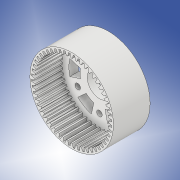
# Autodesk Inventor part: Basespline
Saved by Autodesk Inventor 2017 SP1 (Build 210196100, 196)
## iProperties
Created: 2017-07-11
Part Number: Basespline
Material: ABS Plastic
Document SubType Name: Modeling
Designer: zallen
Density: 1.06 g/cm^3
Appearance: CR White
Author: zallen
Autodesk Inventor part; units mm, degrees
ref_plane "YZ Plane" through (0, 0, 0) normal (1, 0, 0) x (0, 1, 0)
ref_plane "XZ Plane" through (0, 0, 0) normal (0, 1, 0) x (-1, 0, 0)
ref_plane "XY Plane" through (0, 0, 0) normal (0, 0, 1) x (1, 0, 0)
sketch "Sketch1" plane through (0, 0, 0) normal (0, 0, 1) x (1, 0, 0)
  circle A0 centre (0, 0) radius 30 construction
  circle A1 centre (0, 0) radius 33 construction
  circle A2 centre (0, 0) radius 33.1 construction
  circle A3 centre (0, 0) radius 36.1
  line L0 (0, 0) -> (73.8871, 0) construction
  circle A4 centre (0, 0) radius 37.5
  arc A5 (33.0946, -0.6) -> (36.0728, -1.4) centre (38.4543, 13.4097) ccw
  arc A6 (33.0946, 0.6) -> (33.0946, -0.6) centre (53.0856, 0) ccw
  arc A7 (36.0728, 1.4) -> (33.0946, 0.6) centre (38.4543, -13.4097) ccw
  arc A8 (36.0728, -1.4) -> (36.0728, 1.4) centre (0, 0) ccw
  circle A9 centre (0, 0) radius 36.1
  arc A10 (32.9256, 3.3935) -> (35.9786, 2.9583) centre (36.5576, 17.9471) ccw
  arc A11 (35.6411, 5.7379) -> (32.7809, 4.5847) centre (39.7903, -8.6768) ccw
  arc A12 (35.9786, 2.9583) -> (35.6411, 5.7379) centre (0, 0) ccw
  arc A13 (32.7809, 4.5847) -> (32.9256, 3.3935) centre (52.6985, 6.3988) ccw
  circle A14 centre (0, 0) radius 36.1
  arc A15 (32.2765, 7.3375) -> (35.3597, 7.2735) centre (34.1277, 22.2228) ccw
  arc A16 (34.6896, 9.9921) -> (31.9893, 8.5026) centre (40.5461, -3.8174) ccw
  arc A17 (35.3597, 7.2735) -> (34.6896, 9.9921) centre (0, 0) ccw
  arc A18 (31.9893, 8.5026) -> (32.2765, 7.3375) centre (51.543, 12.7042) ccw
  circle A19 centre (0, 0) radius 36.1
  arc A20 (31.1567, 11.1745) -> (34.2251, 11.4826) centre (31.2003, 26.1744) ccw
  arc A21 (33.2322, 14.1006) -> (30.7312, 12.2965) centre (40.7106, 1.0978) ccw
  arc A22 (34.2251, 11.4826) -> (33.2322, 14.1006) centre (0, 0) ccw
  arc A23 (30.7312, 12.2965) -> (31.1567, 11.1745) centre (49.6359, 18.8244) ccw
  circle A24 centre (0, 0) radius 36.1
  arc A25 (29.5826, 14.8485) -> (32.5915, 15.5242) centre (27.8178, 29.7444) ccw
  arc A26 (31.2903, 18.0035) -> (29.0249, 15.9111) centre (40.2814, 5.9969) ccw
  arc A27 (32.5915, 15.5242) -> (31.2903, 18.0035) centre (0, 0) ccw
  arc A28 (29.0249, 15.9111) -> (29.5826, 14.8485) centre (47.0049, 24.6701) ccw
  circle A29 centre (0, 0) radius 36.1
  arc A30 (27.5771, 18.3061) -> (30.4827, 19.3395) centre (24.0297, 32.8805) ccw
  arc A31 (28.8921, 21.6439) -> (26.8955, 19.2936) centre (39.2649, 10.8085) ccw
  arc A32 (30.4827, 19.3395) -> (28.8921, 21.6439) centre (0, 0) ccw
  arc A33 (26.8955, 19.2936) -> (27.5771, 18.3061) centre (43.6886, 30.156) ccw
  circle A34 centre (0, 0) radius 36.1
  arc A35 (25.1695, 21.4966) -> (27.9293, 22.8728) centre (19.8912, 35.5373) ccw
  arc A36 (26.0725, 24.9686) -> (24.3738, 22.3949) centre (37.6758, 15.4626) ccw
  arc A37 (27.9293, 22.8728) -> (26.0725, 24.9686) centre (0, 0) ccw
  arc A38 (24.3738, 22.3949) -> (25.1695, 21.4966) centre (39.7351, 35.2022) ccw
  circle A39 centre (0, 0) radius 36.1
  arc A40 (22.3949, 24.3738) -> (24.9686, 26.0725) centre (15.4626, 37.6758) ccw
  arc A41 (22.8728, 27.9293) -> (21.4966, 25.1695) centre (35.5373, 19.8912) ccw
  arc A42 (24.9686, 26.0725) -> (22.8728, 27.9293) centre (0, 0) ccw
  arc A43 (21.4966, 25.1695) -> (22.3949, 24.3738) centre (35.2022, 39.7351) ccw
  circle A44 centre (0, 0) radius 36.1
  arc A45 (19.2936, 26.8955) -> (21.6439, 28.8921) centre (10.8085, 39.2649) ccw
  arc A46 (19.3395, 30.4827) -> (18.3061, 27.5771) centre (32.8805, 24.0297) ccw
  arc A47 (21.6439, 28.8921) -> (19.3395, 30.4827) centre (0, 0) ccw
  arc A48 (18.3061, 27.5771) -> (19.2936, 26.8955) centre (30.156, 43.6886) ccw
  circle A49 centre (0, 0) radius 36.1
  arc A50 (15.9111, 29.0249) -> (18.0035, 31.2903) centre (5.9969, 40.2814) ccw
  arc A51 (15.5242, 32.5915) -> (14.8485, 29.5826) centre (29.7444, 27.8178) ccw
  arc A52 (18.0035, 31.2903) -> (15.5242, 32.5915) centre (0, 0) ccw
  arc A53 (14.8485, 29.5826) -> (15.9111, 29.0249) centre (24.6701, 47.0049) ccw
  circle A54 centre (0, 0) radius 36.1
  arc A55 (12.2965, 30.7312) -> (14.1006, 33.2322) centre (1.0978, 40.7106) ccw
  arc A56 (11.4826, 34.2251) -> (11.1745, 31.1567) centre (26.1744, 31.2003) ccw
  arc A57 (14.1006, 33.2322) -> (11.4826, 34.2251) centre (0, 0) ccw
  arc A58 (11.1745, 31.1567) -> (12.2965, 30.7312) centre (18.8244, 49.6359) ccw
  circle A59 centre (0, 0) radius 36.1
  arc A60 (8.5026, 31.9893) -> (9.9921, 34.6896) centre (-3.8174, 40.5461) ccw
  arc A61 (7.2735, 35.3597) -> (7.3375, 32.2765) centre (22.2228, 34.1277) ccw
  arc A62 (9.9921, 34.6896) -> (7.2735, 35.3597) centre (0, 0) ccw
  arc A63 (7.3375, 32.2765) -> (8.5026, 31.9893) centre (12.7042, 51.543) ccw
  circle A64 centre (0, 0) radius 36.1
  arc A65 (4.5847, 32.7809) -> (5.7379, 35.6411) centre (-8.6768, 39.7903) ccw
  arc A66 (2.9583, 35.9786) -> (3.3935, 32.9256) centre (17.9471, 36.5576) ccw
  arc A67 (5.7379, 35.6411) -> (2.9583, 35.9786) centre (0, 0) ccw
  arc A68 (3.3935, 32.9256) -> (4.5847, 32.7809) centre (6.3988, 52.6985) ccw
  circle A69 centre (0, 0) radius 36.1
  arc A70 (0.6, 33.0946) -> (1.4, 36.0728) centre (-13.4097, 38.4543) ccw
  arc A71 (-1.4, 36.0728) -> (-0.6, 33.0946) centre (13.4097, 38.4543) ccw
  arc A72 (1.4, 36.0728) -> (-1.4, 36.0728) centre (0, 0) ccw
  arc A73 (-0.6, 33.0946) -> (0.6, 33.0946) centre (0, 53.0856) ccw
  circle A74 centre (0, 0) radius 36.1
  arc A75 (-3.3935, 32.9256) -> (-2.9583, 35.9786) centre (-17.9471, 36.5576) ccw
  arc A76 (-5.7379, 35.6411) -> (-4.5847, 32.7809) centre (8.6768, 39.7903) ccw
  arc A77 (-2.9583, 35.9786) -> (-5.7379, 35.6411) centre (0, 0) ccw
  arc A78 (-4.5847, 32.7809) -> (-3.3935, 32.9256) centre (-6.3988, 52.6985) ccw
  circle A79 centre (0, 0) radius 36.1
  arc A80 (-7.3375, 32.2765) -> (-7.2735, 35.3597) centre (-22.2228, 34.1277) ccw
  arc A81 (-9.9921, 34.6896) -> (-8.5026, 31.9893) centre (3.8174, 40.5461) ccw
  arc A82 (-7.2735, 35.3597) -> (-9.9921, 34.6896) centre (0, 0) ccw
  arc A83 (-8.5026, 31.9893) -> (-7.3375, 32.2765) centre (-12.7042, 51.543) ccw
  circle A84 centre (0, 0) radius 36.1
  arc A85 (-11.1745, 31.1567) -> (-11.4826, 34.2251) centre (-26.1744, 31.2003) ccw
  arc A86 (-14.1006, 33.2322) -> (-12.2965, 30.7312) centre (-1.0978, 40.7106) ccw
  arc A87 (-11.4826, 34.2251) -> (-14.1006, 33.2322) centre (0, 0) ccw
  arc A88 (-12.2965, 30.7312) -> (-11.1745, 31.1567) centre (-18.8244, 49.6359) ccw
  circle A89 centre (0, 0) radius 36.1
  arc A90 (-14.8485, 29.5826) -> (-15.5242, 32.5915) centre (-29.7444, 27.8178) ccw
  arc A91 (-18.0035, 31.2903) -> (-15.9111, 29.0249) centre (-5.9969, 40.2814) ccw
  arc A92 (-15.5242, 32.5915) -> (-18.0035, 31.2903) centre (0, 0) ccw
  arc A93 (-15.9111, 29.0249) -> (-14.8485, 29.5826) centre (-24.6701, 47.0049) ccw
  circle A94 centre (0, 0) radius 36.1
  arc A95 (-18.3061, 27.5771) -> (-19.3395, 30.4827) centre (-32.8805, 24.0297) ccw
  arc A96 (-21.6439, 28.8921) -> (-19.2936, 26.8955) centre (-10.8085, 39.2649) ccw
  arc A97 (-19.3395, 30.4827) -> (-21.6439, 28.8921) centre (0, 0) ccw
  arc A98 (-19.2936, 26.8955) -> (-18.3061, 27.5771) centre (-30.156, 43.6886) ccw
  circle A99 centre (0, 0) radius 36.1
  arc A100 (-21.4966, 25.1695) -> (-22.8728, 27.9293) centre (-35.5373, 19.8912) ccw
  arc A101 (-24.9686, 26.0725) -> (-22.3949, 24.3738) centre (-15.4626, 37.6758) ccw
  arc A102 (-22.8728, 27.9293) -> (-24.9686, 26.0725) centre (0, 0) ccw
  arc A103 (-22.3949, 24.3738) -> (-21.4966, 25.1695) centre (-35.2022, 39.7351) ccw
  circle A104 centre (0, 0) radius 36.1
  arc A105 (-24.3738, 22.3949) -> (-26.0725, 24.9686) centre (-37.6758, 15.4626) ccw
  arc A106 (-27.9293, 22.8728) -> (-25.1695, 21.4966) centre (-19.8912, 35.5373) ccw
  arc A107 (-26.0725, 24.9686) -> (-27.9293, 22.8728) centre (0, 0) ccw
  arc A108 (-25.1695, 21.4966) -> (-24.3738, 22.3949) centre (-39.7351, 35.2022) ccw
  circle A109 centre (0, 0) radius 36.1
  arc A110 (-26.8955, 19.2936) -> (-28.8921, 21.6439) centre (-39.2649, 10.8085) ccw
  arc A111 (-30.4827, 19.3395) -> (-27.5771, 18.3061) centre (-24.0297, 32.8805) ccw
  arc A112 (-28.8921, 21.6439) -> (-30.4827, 19.3395) centre (0, 0) ccw
  arc A113 (-27.5771, 18.3061) -> (-26.8955, 19.2936) centre (-43.6886, 30.156) ccw
  circle A114 centre (0, 0) radius 36.1
  arc A115 (-29.0249, 15.9111) -> (-31.2903, 18.0035) centre (-40.2814, 5.9969) ccw
  arc A116 (-32.5915, 15.5242) -> (-29.5826, 14.8485) centre (-27.8178, 29.7444) ccw
  arc A117 (-31.2903, 18.0035) -> (-32.5915, 15.5242) centre (0, 0) ccw
  arc A118 (-29.5826, 14.8485) -> (-29.0249, 15.9111) centre (-47.0049, 24.6701) ccw
  circle A119 centre (0, 0) radius 36.1
  arc A120 (-30.7312, 12.2965) -> (-33.2322, 14.1006) centre (-40.7106, 1.0978) ccw
  arc A121 (-34.2251, 11.4826) -> (-31.1567, 11.1745) centre (-31.2003, 26.1744) ccw
  arc A122 (-33.2322, 14.1006) -> (-34.2251, 11.4826) centre (0, 0) ccw
  arc A123 (-31.1567, 11.1745) -> (-30.7312, 12.2965) centre (-49.6359, 18.8244) ccw
  circle A124 centre (0, 0) radius 36.1
  arc A125 (-31.9893, 8.5026) -> (-34.6896, 9.9921) centre (-40.5461, -3.8174) ccw
  arc A126 (-35.3597, 7.2735) -> (-32.2765, 7.3375) centre (-34.1277, 22.2228) ccw
  arc A127 (-34.6896, 9.9921) -> (-35.3597, 7.2735) centre (0, 0) ccw
  arc A128 (-32.2765, 7.3375) -> (-31.9893, 8.5026) centre (-51.543, 12.7042) ccw
  circle A129 centre (0, 0) radius 36.1
  arc A130 (-32.7809, 4.5847) -> (-35.6411, 5.7379) centre (-39.7903, -8.6768) ccw
  arc A131 (-35.9786, 2.9583) -> (-32.9256, 3.3935) centre (-36.5576, 17.9471) ccw
  arc A132 (-35.6411, 5.7379) -> (-35.9786, 2.9583) centre (0, 0) ccw
  arc A133 (-32.9256, 3.3935) -> (-32.7809, 4.5847) centre (-52.6985, 6.3988) ccw
  circle A134 centre (0, 0) radius 36.1
  arc A135 (-33.0946, 0.6) -> (-36.0728, 1.4) centre (-38.4543, -13.4097) ccw
  arc A136 (-36.0728, -1.4) -> (-33.0946, -0.6) centre (-38.4543, 13.4097) ccw
  arc A137 (-36.0728, 1.4) -> (-36.0728, -1.4) centre (0, 0) ccw
  arc A138 (-33.0946, -0.6) -> (-33.0946, 0.6) centre (-53.0856, 0) ccw
  circle A139 centre (0, 0) radius 36.1
  arc A140 (-32.9256, -3.3935) -> (-35.9786, -2.9583) centre (-36.5576, -17.9471) ccw
  arc A141 (-35.6411, -5.7379) -> (-32.7809, -4.5847) centre (-39.7903, 8.6768) ccw
  arc A142 (-35.9786, -2.9583) -> (-35.6411, -5.7379) centre (0, 0) ccw
  arc A143 (-32.7809, -4.5847) -> (-32.9256, -3.3935) centre (-52.6985, -6.3988) ccw
  circle A144 centre (0, 0) radius 36.1
  arc A145 (-32.2765, -7.3375) -> (-35.3597, -7.2735) centre (-34.1277, -22.2228) ccw
  arc A146 (-34.6896, -9.9921) -> (-31.9893, -8.5026) centre (-40.5461, 3.8174) ccw
  arc A147 (-35.3597, -7.2735) -> (-34.6896, -9.9921) centre (0, 0) ccw
  arc A148 (-31.9893, -8.5026) -> (-32.2765, -7.3375) centre (-51.543, -12.7042) ccw
  circle A149 centre (0, 0) radius 36.1
  arc A150 (-31.1567, -11.1745) -> (-34.2251, -11.4826) centre (-31.2003, -26.1744) ccw
  arc A151 (-33.2322, -14.1006) -> (-30.7312, -12.2965) centre (-40.7106, -1.0978) ccw
  arc A152 (-34.2251, -11.4826) -> (-33.2322, -14.1006) centre (0, 0) ccw
  arc A153 (-30.7312, -12.2965) -> (-31.1567, -11.1745) centre (-49.6359, -18.8244) ccw
  circle A154 centre (0, 0) radius 36.1
  arc A155 (-29.5826, -14.8485) -> (-32.5915, -15.5242) centre (-27.8178, -29.7444) ccw
  arc A156 (-31.2903, -18.0035) -> (-29.0249, -15.9111) centre (-40.2814, -5.9969) ccw
  arc A157 (-32.5915, -15.5242) -> (-31.2903, -18.0035) centre (0, 0) ccw
  arc A158 (-29.0249, -15.9111) -> (-29.5826, -14.8485) centre (-47.0049, -24.6701) ccw
  circle A159 centre (0, 0) radius 36.1
  arc A160 (-27.5771, -18.3061) -> (-30.4827, -19.3395) centre (-24.0297, -32.8805) ccw
  arc A161 (-28.8921, -21.6439) -> (-26.8955, -19.2936) centre (-39.2649, -10.8085) ccw
  arc A162 (-30.4827, -19.3395) -> (-28.8921, -21.6439) centre (0, 0) ccw
  arc A163 (-26.8955, -19.2936) -> (-27.5771, -18.3061) centre (-43.6886, -30.156) ccw
  circle A164 centre (0, 0) radius 36.1
  arc A165 (-25.1695, -21.4966) -> (-27.9293, -22.8728) centre (-19.8912, -35.5373) ccw
  arc A166 (-26.0725, -24.9686) -> (-24.3738, -22.3949) centre (-37.6758, -15.4626) ccw
  arc A167 (-27.9293, -22.8728) -> (-26.0725, -24.9686) centre (0, 0) ccw
  arc A168 (-24.3738, -22.3949) -> (-25.1695, -21.4966) centre (-39.7351, -35.2022) ccw
  circle A169 centre (0, 0) radius 36.1
  arc A170 (-22.3949, -24.3738) -> (-24.9686, -26.0725) centre (-15.4626, -37.6758) ccw
  arc A171 (-22.8728, -27.9293) -> (-21.4966, -25.1695) centre (-35.5373, -19.8912) ccw
  arc A172 (-24.9686, -26.0725) -> (-22.8728, -27.9293) centre (0, 0) ccw
  arc A173 (-21.4966, -25.1695) -> (-22.3949, -24.3738) centre (-35.2022, -39.7351) ccw
  circle A174 centre (0, 0) radius 36.1
  arc A175 (-19.2936, -26.8955) -> (-21.6439, -28.8921) centre (-10.8085, -39.2649) ccw
  arc A176 (-19.3395, -30.4827) -> (-18.3061, -27.5771) centre (-32.8805, -24.0297) ccw
  arc A177 (-21.6439, -28.8921) -> (-19.3395, -30.4827) centre (0, 0) ccw
  arc A178 (-18.3061, -27.5771) -> (-19.2936, -26.8955) centre (-30.156, -43.6886) ccw
  circle A179 centre (0, 0) radius 36.1
  arc A180 (-15.9111, -29.0249) -> (-18.0035, -31.2903) centre (-5.9969, -40.2814) ccw
  arc A181 (-15.5242, -32.5915) -> (-14.8485, -29.5826) centre (-29.7444, -27.8178) ccw
  arc A182 (-18.0035, -31.2903) -> (-15.5242, -32.5915) centre (0, 0) ccw
  arc A183 (-14.8485, -29.5826) -> (-15.9111, -29.0249) centre (-24.6701, -47.0049) ccw
  circle A184 centre (0, 0) radius 36.1
  arc A185 (-12.2965, -30.7312) -> (-14.1006, -33.2322) centre (-1.0978, -40.7106) ccw
  arc A186 (-11.4826, -34.2251) -> (-11.1745, -31.1567) centre (-26.1744, -31.2003) ccw
  arc A187 (-14.1006, -33.2322) -> (-11.4826, -34.2251) centre (0, 0) ccw
  arc A188 (-11.1745, -31.1567) -> (-12.2965, -30.7312) centre (-18.8244, -49.6359) ccw
  circle A189 centre (0, 0) radius 36.1
  arc A190 (-8.5026, -31.9893) -> (-9.9921, -34.6896) centre (3.8174, -40.5461) ccw
  arc A191 (-7.2735, -35.3597) -> (-7.3375, -32.2765) centre (-22.2228, -34.1277) ccw
  arc A192 (-9.9921, -34.6896) -> (-7.2735, -35.3597) centre (0, 0) ccw
  arc A193 (-7.3375, -32.2765) -> (-8.5026, -31.9893) centre (-12.7042, -51.543) ccw
  circle A194 centre (0, 0) radius 36.1
  arc A195 (-4.5847, -32.7809) -> (-5.7379, -35.6411) centre (8.6768, -39.7903) ccw
  arc A196 (-2.9583, -35.9786) -> (-3.3935, -32.9256) centre (-17.9471, -36.5576) ccw
  arc A197 (-5.7379, -35.6411) -> (-2.9583, -35.9786) centre (0, 0) ccw
  arc A198 (-3.3935, -32.9256) -> (-4.5847, -32.7809) centre (-6.3988, -52.6985) ccw
  circle A199 centre (0, 0) radius 36.1
  arc A200 (-0.6, -33.0946) -> (-1.4, -36.0728) centre (13.4097, -38.4543) ccw
  arc A201 (1.4, -36.0728) -> (0.6, -33.0946) centre (-13.4097, -38.4543) ccw
  arc A202 (-1.4, -36.0728) -> (1.4, -36.0728) centre (0, 0) ccw
  arc A203 (0.6, -33.0946) -> (-0.6, -33.0946) centre (0, -53.0856) ccw
  circle A204 centre (0, 0) radius 36.1
  arc A205 (3.3935, -32.9256) -> (2.9583, -35.9786) centre (17.9471, -36.5576) ccw
  arc A206 (5.7379, -35.6411) -> (4.5847, -32.7809) centre (-8.6768, -39.7903) ccw
  arc A207 (2.9583, -35.9786) -> (5.7379, -35.6411) centre (0, 0) ccw
  arc A208 (4.5847, -32.7809) -> (3.3935, -32.9256) centre (6.3988, -52.6985) ccw
  circle A209 centre (0, 0) radius 36.1
  arc A210 (7.3375, -32.2765) -> (7.2735, -35.3597) centre (22.2228, -34.1277) ccw
  arc A211 (9.9921, -34.6896) -> (8.5026, -31.9893) centre (-3.8174, -40.5461) ccw
  arc A212 (7.2735, -35.3597) -> (9.9921, -34.6896) centre (0, 0) ccw
  arc A213 (8.5026, -31.9893) -> (7.3375, -32.2765) centre (12.7042, -51.543) ccw
  circle A214 centre (0, 0) radius 36.1
  arc A215 (11.1745, -31.1567) -> (11.4826, -34.2251) centre (26.1744, -31.2003) ccw
  arc A216 (14.1006, -33.2322) -> (12.2965, -30.7312) centre (1.0978, -40.7106) ccw
  arc A217 (11.4826, -34.2251) -> (14.1006, -33.2322) centre (0, 0) ccw
  arc A218 (12.2965, -30.7312) -> (11.1745, -31.1567) centre (18.8244, -49.6359) ccw
  circle A219 centre (0, 0) radius 36.1
  arc A220 (14.8485, -29.5826) -> (15.5242, -32.5915) centre (29.7444, -27.8178) ccw
  arc A221 (18.0035, -31.2903) -> (15.9111, -29.0249) centre (5.9969, -40.2814) ccw
  arc A222 (15.5242, -32.5915) -> (18.0035, -31.2903) centre (0, 0) ccw
  arc A223 (15.9111, -29.0249) -> (14.8485, -29.5826) centre (24.6701, -47.0049) ccw
  circle A224 centre (0, 0) radius 36.1
  arc A225 (18.3061, -27.5771) -> (19.3395, -30.4827) centre (32.8805, -24.0297) ccw
  arc A226 (21.6439, -28.8921) -> (19.2936, -26.8955) centre (10.8085, -39.2649) ccw
  arc A227 (19.3395, -30.4827) -> (21.6439, -28.8921) centre (0, 0) ccw
  arc A228 (19.2936, -26.8955) -> (18.3061, -27.5771) centre (30.156, -43.6886) ccw
  circle A229 centre (0, 0) radius 36.1
  arc A230 (21.4966, -25.1695) -> (22.8728, -27.9293) centre (35.5373, -19.8912) ccw
  arc A231 (24.9686, -26.0725) -> (22.3949, -24.3738) centre (15.4626, -37.6758) ccw
  arc A232 (22.8728, -27.9293) -> (24.9686, -26.0725) centre (0, 0) ccw
  arc A233 (22.3949, -24.3738) -> (21.4966, -25.1695) centre (35.2022, -39.7351) ccw
  circle A234 centre (0, 0) radius 36.1
  arc A235 (24.3738, -22.3949) -> (26.0725, -24.9686) centre (37.6758, -15.4626) ccw
  arc A236 (27.9293, -22.8728) -> (25.1695, -21.4966) centre (19.8912, -35.5373) ccw
  arc A237 (26.0725, -24.9686) -> (27.9293, -22.8728) centre (0, 0) ccw
  arc A238 (25.1695, -21.4966) -> (24.3738, -22.3949) centre (39.7351, -35.2022) ccw
  circle A239 centre (0, 0) radius 36.1
  arc A240 (26.8955, -19.2936) -> (28.8921, -21.6439) centre (39.2649, -10.8085) ccw
  arc A241 (30.4827, -19.3395) -> (27.5771, -18.3061) centre (24.0297, -32.8805) ccw
  arc A242 (28.8921, -21.6439) -> (30.4827, -19.3395) centre (0, 0) ccw
  arc A243 (27.5771, -18.3061) -> (26.8955, -19.2936) centre (43.6886, -30.156) ccw
  circle A244 centre (0, 0) radius 36.1
  arc A245 (29.0249, -15.9111) -> (31.2903, -18.0035) centre (40.2814, -5.9969) ccw
  arc A246 (32.5915, -15.5242) -> (29.5826, -14.8485) centre (27.8178, -29.7444) ccw
  arc A247 (31.2903, -18.0035) -> (32.5915, -15.5242) centre (0, 0) ccw
  arc A248 (29.5826, -14.8485) -> (29.0249, -15.9111) centre (47.0049, -24.6701) ccw
  circle A249 centre (0, 0) radius 36.1
  arc A250 (30.7312, -12.2965) -> (33.2322, -14.1006) centre (40.7106, -1.0978) ccw
  arc A251 (34.2251, -11.4826) -> (31.1567, -11.1745) centre (31.2003, -26.1744) ccw
  arc A252 (33.2322, -14.1006) -> (34.2251, -11.4826) centre (0, 0) ccw
  arc A253 (31.1567, -11.1745) -> (30.7312, -12.2965) centre (49.6359, -18.8244) ccw
  circle A254 centre (0, 0) radius 36.1
  arc A255 (31.9893, -8.5026) -> (34.6896, -9.9921) centre (40.5461, 3.8174) ccw
  arc A256 (35.3597, -7.2735) -> (32.2765, -7.3375) centre (34.1277, -22.2228) ccw
  arc A257 (34.6896, -9.9921) -> (35.3597, -7.2735) centre (0, 0) ccw
  arc A258 (32.2765, -7.3375) -> (31.9893, -8.5026) centre (51.543, -12.7042) ccw
  circle A259 centre (0, 0) radius 36.1
  arc A260 (32.7809, -4.5847) -> (35.6411, -5.7379) centre (39.7903, 8.6768) ccw
  arc A261 (35.9786, -2.9583) -> (32.9256, -3.3935) centre (36.5576, -17.9471) ccw
  arc A262 (35.6411, -5.7379) -> (35.9786, -2.9583) centre (0, 0) ccw
  arc A263 (32.9256, -3.3935) -> (32.7809, -4.5847) centre (52.6985, -6.3988) ccw
  point P0 (33.0856, 0)
  point P1 (32.8443, 3.988)
  point P2 (32.1242, 7.9179)
  point P3 (30.9355, 11.7323)
  point P4 (29.2958, 15.3756)
  point P5 (27.2289, 18.7947)
  point P6 (24.7649, 21.9398)
  point P7 (21.9398, 24.7649)
  point P8 (18.7947, 27.2289)
  point P9 (15.3756, 29.2958)
  point P10 (11.7323, 30.9355)
  point P11 (7.9179, 32.1242)
  point P12 (3.988, 32.8443)
  point P13 (0, 33.0856)
  point P14 (-3.988, 32.8443)
  point P15 (-7.9179, 32.1242)
  point P16 (-11.7323, 30.9355)
  point P17 (-15.3756, 29.2958)
  point P18 (-18.7947, 27.2289)
  point P19 (-21.9398, 24.7649)
  point P20 (-24.7649, 21.9398)
  point P21 (-27.2289, 18.7947)
  point P22 (-29.2958, 15.3756)
  point P23 (-30.9355, 11.7323)
  point P24 (-32.1242, 7.9179)
  point P25 (-32.8443, 3.988)
  point P26 (-33.0856, 0)
  point P27 (-32.8443, -3.988)
  point P28 (-32.1242, -7.9179)
  point P29 (-30.9355, -11.7323)
  point P30 (-29.2958, -15.3756)
  point P31 (-27.2289, -18.7947)
  point P32 (-24.7649, -21.9398)
  point P33 (-21.9398, -24.7649)
  point P34 (-18.7947, -27.2289)
  point P35 (-15.3756, -29.2958)
  point P36 (-11.7323, -30.9355)
  point P37 (-7.9179, -32.1242)
  point P38 (-3.988, -32.8443)
  point P39 (0, -33.0856)
  point P40 (3.988, -32.8443)
  point P41 (7.9179, -32.1242)
  point P42 (11.7323, -30.9355)
  point P43 (15.3756, -29.2958)
  point P44 (18.7947, -27.2289)
  point P45 (21.9398, -24.7649)
  point P46 (24.7649, -21.9398)
  point P47 (27.2289, -18.7947)
  point P48 (29.2958, -15.3756)
  point P49 (30.9355, -11.7323)
  point P50 (32.1242, -7.9179)
  point P51 (32.8443, -3.988)
  dimension "d0" = 60
  dimension "d1" = 3
  dimension "d2" = 0.1
  dimension "d3" = 3
  dimension "d4" = 75
  dimension "d5" = 15
  dimension "d6" = 20
  dimension "d7" = 1.2
  dimension "d8" = 1.4
  dimension "d15" = 360
  constraints: 419 point on circle, 212 centre point, 4 coincident, 2 end point, 2 symmetric about line, 1 horizontal, 1 point on line, 988 other
  measures "d0" diameter of A0
  measures "d1" radial gap between concentric circles of A0 A1
  measures "d2" radial gap between concentric circles of A1 A2
  measures "d4" diameter of A4
  measures "d5" radius of A5
  measures "d6" radius of A6
  measures "d7" distance of A2.end A2.start
  measures "d8" distance from line of L0 A5.end
extrude "Extrusion1" add sketch "Sketch1" along normal blind 25 contours A3 A5 A6 A7 | A10 A13 A11 A3 | A3 A260 A263 A261 | A15 A18 A16 A3 | A3 A255 A258 A256 | A20 A23 A21 A3 | A3 A250 A253 A251 | A25 A28 A26 A3 | A3 A245 A248 A246 | A30 A33 A31 A3 | A3 A240 A243 A241 | A35 A38 A36 A3 | A3 A235 A238 A236 | A40 A43 A41 A3 | A3 A230 A233 A231 | A45 A48 A46 A3 | A3 A225 A228 A226 | A50 A53 A51 A3 | A3 A220 A223 A221 | A55 A58 A56 A3 | A3 A215 A218 A216 | A60 A63 A61 A3 | A3 A210 A213 A211 | A65 A68 A66 A3 | A3 A205 A208 A206 | A70 A73 A71 A3 | A3 A200 A203 A201 | A75 A78 A76 A3 | A3 A195 A198 A196 | A80 A83 A81 A3 | A3 A190 A193 A191 | A85 A88 A86 A3 | A3 A185 A188 A186 | A90 A93 A91 A3 | A3 A180 A183 A181 | A95 A98 A96 A3 | A3 A175 A178 A176 | A100 A103 A101 A3 | A3 A170 A173 A171 | A105 A108 A106 A3 | A3 A165 A168 A166 | A110 A113 A111 A3 | A3 A160 A163 A161 | A115 A118 A116 A3 | A3 A155 A158 A156 | A120 A123 A121 A3 | A3 A150 A153 A151 | A125 A128 A126 A3 | A3 A145 A148 A146 | A130 A133 A131 A3 | A3 A140 A143 A141 | A135 A138 A136 A3 | A4
sketch "Sketch2" plane through (0, 0, 0) normal (0, 0, -1) x (-1, 0, 0)
  circle A0 centre (0, 0) radius 37.5 projected
  circle A1 centre (0, 0) radius 11
  circle A2 centre (0, 0) radius 27.5 construction
  line L0 (26.5942, 7) -> (17.0367, 4)
  line L1 (26.5942, -7) -> (17.0367, -4)
  arc A3 (17.0367, -4) -> (17.0367, 4) centre (0, 0) ccw
  arc A4 (26.5942, -7) -> (26.5942, 7) centre (0, 0) ccw
  circle A5 centre (0, 0) radius 17.5 construction
  line L2 (7.2349, 26.5312) -> (5.0543, 16.7542)
  arc A6 (11.9825, 12.7542) -> (5.0543, 16.7542) centre (0, 0) ccw
  line L3 (19.3593, 19.5312) -> (11.9825, 12.7542)
  circle A7 centre (0, 0) radius 27.5 construction
  arc A8 (19.3593, 19.5312) -> (7.2349, 26.5312) centre (0, 0) ccw
  line L4 (-19.3593, 19.5312) -> (-11.9825, 12.7542)
  arc A9 (-5.0543, 16.7542) -> (-11.9825, 12.7542) centre (0, 0) ccw
  line L5 (-7.2349, 26.5312) -> (-5.0543, 16.7542)
  circle A10 centre (0, 0) radius 27.5 construction
  arc A11 (-7.2349, 26.5312) -> (-19.3593, 19.5312) centre (0, 0) ccw
  line L6 (-26.5942, -7) -> (-17.0367, -4)
  arc A12 (-17.0367, 4) -> (-17.0367, -4) centre (0, 0) ccw
  line L7 (-26.5942, 7) -> (-17.0367, 4)
  circle A13 centre (0, 0) radius 27.5 construction
  arc A14 (-26.5942, 7) -> (-26.5942, -7) centre (0, 0) ccw
  line L8 (-7.2349, -26.5312) -> (-5.0543, -16.7542)
  arc A15 (-11.9825, -12.7542) -> (-5.0543, -16.7542) centre (0, 0) ccw
  line L9 (-19.3593, -19.5312) -> (-11.9825, -12.7542)
  circle A16 centre (0, 0) radius 27.5 construction
  arc A17 (-19.3593, -19.5312) -> (-7.2349, -26.5312) centre (0, 0) ccw
  line L10 (19.3593, -19.5312) -> (11.9825, -12.7542)
  arc A18 (5.0543, -16.7542) -> (11.9825, -12.7542) centre (0, 0) ccw
  line L11 (7.2349, -26.5312) -> (5.0543, -16.7542)
  circle A19 centre (0, 0) radius 27.5 construction
  arc A20 (7.2349, -26.5312) -> (19.3593, -19.5312) centre (0, 0) ccw
  circle A21 centre (0, 0) radius 22.5 construction
  circle A22 centre (19.4856, -11.25) radius 2.5
  line L12 (21.8173, -5.5006) -> (15.6723, -16.144) construction
  line L13 (18.7448, -10.8223) -> (19.4856, -11.25) construction
  circle A23 centre (19.4856, 11.25) radius 2.5
  circle A24 centre (0, 22.5) radius 2.5
  circle A25 centre (-19.4856, 11.25) radius 2.5
  circle A26 centre (-19.4856, -11.25) radius 2.5
  circle A27 centre (0, -22.5) radius 2.5
  point P0 (17.5, 0)
  point P1 (27.5, 0)
  point P2 (8.75, 15.1554)
  point P3 (13.75, 23.8157)
  point P4 (-8.75, 15.1554)
  point P5 (-13.75, 23.8157)
  point P6 (-17.5, 0)
  point P7 (-27.5, 0)
  point P8 (-8.75, -15.1554)
  point P9 (-13.75, -23.8157)
  point P10 (8.75, -15.1554)
  point P11 (13.75, -23.8157)
  dimension "d21" = 55
  dimension "d35" = 35
  dimension "d19" = 22
  dimension "d22" = 7
  dimension "d23" = 4
  dimension "d32" = 7
  dimension "d33" = 4
  dimension "d42" = 360
  dimension "d46" = 45
  dimension "d47" = 5
  dimension "d48" = 90
  dimension "d51" = 360
  constraints: 29 point on circle, 28 end point, 20 centre point, 10 coincident, 2 point on line, 1 midpoint, 126 other
  measures "d19" diameter of A1
  measures "d22" vertical distance of point (0, 0) L0.start
  measures "d23" vertical distance of point (0, 0) L0.end
  measures "d32" vertical distance of L1.start point (27.5, 0)
  measures "d33" vertical distance of point (0, 0) L1.end
  measures "d46" diameter of A21
  measures "d47" diameter of A22
  measures "d48" angle of L12 L13
extrude "Extrusion2" add sketch "Sketch2" along normal blind 8
body "Solid1"
